Autodesk Fusion 360 part; units mm, degrees
note: some values were not read from the file. Set by a fixed rule: which sketch regions a step uses.
(part 2 of 2)
sketch "Sketch3" plane through (0, 0, 4.699) normal (0, 0, 1) x (-1, 0, 0)
  line L0 (-146.1673, -221.1104) -> (-150.3628, -221.1104)
  line L1 (-150.3628, -221.1104) -> (-150.3628, -216.6156)
  line L2 (-150.3628, -216.6156) -> (-146.1673, -216.6156)
  line L3 (-146.1673, -216.6156) -> (-146.1673, -221.1104)
  line L4 (-156.9944, -229.4223) -> (-156.9944, -223.3483)
  line L5 (-156.9944, -223.3483) -> (-152.6466, -223.3483)
  line L6 (-152.6466, -223.3483) -> (-152.6466, -229.4223)
  line L7 (-152.6466, -229.4223) -> (-156.9944, -229.4223)
  line L8 (-170.3485, -221.1104) -> (-170.3485, -216.6156)
  line L9 (-170.3485, -216.6156) -> (-165.8649, -216.6156)
  line L10 (-165.8649, -216.6156) -> (-165.8649, -221.1104)
  line L11 (-165.8649, -221.1104) -> (-170.3485, -221.1104)
  line L12 (-180.9883, -210.0039) -> (-180.9883, -214.3606)
  line L13 (-180.9883, -214.3606) -> (-183.4799, -214.3606)
  line L14 (-183.4799, -214.3606) -> (-181.7379, -210.0039)
  line L15 (-181.7379, -210.0039) -> (-180.9883, -210.0039)
  line L16 (-156.9944, -233.3153) -> (-156.9944, -231.7356)
  line L17 (-156.9944, -231.7356) -> (-154.4457, -231.7356)
  line L18 (-154.4457, -231.7356) -> (-156.9944, -233.3153)
  line L19 (-150.3628, -223.3483) -> (-146.1673, -223.3483)
  line L20 (-146.1673, -223.3483) -> (-146.1673, -226.6039)
  line L21 (-146.1673, -226.6039) -> (-150.3628, -229.2048)
  line L22 (-150.3628, -229.2048) -> (-150.3628, -223.3483)
  line L23 (-152.6466, -207.7364) -> (-156.9944, -207.7364)
  line L24 (-156.9944, -207.7364) -> (-156.9944, -203.394)
  line L25 (-156.9944, -203.394) -> (-152.6466, -203.394)
  line L26 (-152.6466, -203.394) -> (-152.6466, -207.7364)
  line L27 (-143.2758, -207.7364) -> (-143.8532, -207.7364)
  line L28 (-143.8532, -207.7364) -> (-143.8532, -206.2865)
  line L29 (-143.8532, -206.2865) -> (-143.2758, -207.7364)
  line L30 (-163.3746, -235.1382) -> (-163.3746, -231.9856)
  line L31 (-163.3746, -231.9856) -> (-159.447, -231.9856)
  line L32 (-159.447, -231.9856) -> (-159.447, -234.8356)
  line L33 (-159.447, -234.8356) -> (-161.6393, -236.1945)
  line L34 (-161.6393, -236.1945) -> (-163.3746, -235.1382)
  line L35 (-172.6153, -203.394) -> (-172.6153, -207.7364)
  line L36 (-172.6153, -207.7364) -> (-178.675, -207.7364)
  line L37 (-178.675, -207.7364) -> (-178.675, -203.394)
  line L38 (-178.675, -203.394) -> (-172.6153, -203.394)
  line L39 (-163.616, -229.4223) -> (-163.616, -223.3483)
  line L40 (-163.616, -223.3483) -> (-159.2509, -223.3483)
  line L41 (-159.2509, -223.3483) -> (-159.2509, -229.4223)
  line L42 (-159.2509, -229.4223) -> (-163.616, -229.4223)
  line L43 (-165.8649, -190.62) -> (-165.8649, -194.6061)
  line L44 (-165.8649, -194.6061) -> (-170.3485, -194.6061)
  line L45 (-170.3485, -194.6061) -> (-170.3485, -192.7692)
  line L46 (-170.3485, -192.7692) -> (-165.8649, -190.62)
  line L47 (-180.9883, -223.3483) -> (-180.9883, -224.6638)
  line L48 (-180.9883, -224.6638) -> (-183.1496, -223.3483)
  line L49 (-183.1496, -223.3483) -> (-180.9883, -223.3483)
  line L50 (-163.616, -214.3606) -> (-163.616, -210.0039)
  line L51 (-163.616, -210.0039) -> (-159.2509, -210.0039)
  line L52 (-159.2509, -210.0039) -> (-159.2509, -214.3606)
  line L53 (-159.2509, -214.3606) -> (-163.616, -214.3606)
  line L54 (-165.8649, -196.9098) -> (-165.8649, -201.1101)
  line L55 (-165.8649, -201.1101) -> (-170.3485, -201.1101)
  line L56 (-170.3485, -201.1101) -> (-170.3485, -196.9098)
  line L57 (-170.3485, -196.9098) -> (-165.8649, -196.9098)
  line L58 (-180.9883, -208.1294) -> (-180.9883, -208.2364)
  line L59 (-180.9883, -208.2364) -> (-181.031, -208.2364)
  line L60 (-181.031, -208.2364) -> (-180.9883, -208.1294)
  line L61 (-152.6466, -193.2326) -> (-152.6466, -194.6061)
  line L62 (-152.6466, -194.6061) -> (-156.9944, -194.6061)
  line L63 (-156.9944, -194.6061) -> (-156.9944, -191.0845)
  line L64 (-156.9944, -191.0845) -> (-152.6466, -193.2326)
  line L65 (-159.2509, -196.9098) -> (-159.2509, -201.1101)
  line L66 (-159.2509, -201.1101) -> (-163.616, -201.1101)
  line L67 (-163.616, -201.1101) -> (-163.616, -196.9098)
  line L68 (-163.616, -196.9098) -> (-159.2509, -196.9098)
  line L69 (-172.6153, -210.0039) -> (-172.6153, -214.3606)
  line L70 (-172.6153, -214.3606) -> (-178.675, -214.3606)
  line L71 (-178.675, -214.3606) -> (-178.675, -210.0039)
  line L72 (-178.675, -210.0039) -> (-172.6153, -210.0039)
  line L73 (-152.6466, -210.0039) -> (-152.6466, -214.3606)
  line L74 (-152.6466, -214.3606) -> (-156.9944, -214.3606)
  line L75 (-156.9944, -214.3606) -> (-156.9944, -210.0039)
  line L76 (-156.9944, -210.0039) -> (-152.6466, -210.0039)
  line L77 (-165.8649, -203.394) -> (-165.8649, -207.7364)
  line L78 (-165.8649, -207.7364) -> (-170.3485, -207.7364)
  line L79 (-170.3485, -207.7364) -> (-170.3485, -203.394)
  line L80 (-170.3485, -203.394) -> (-165.8649, -203.394)
  line L81 (-159.2509, -194.6061) -> (-163.616, -194.6061)
  line L82 (-163.616, -194.6061) -> (-163.616, -189.5422)
  line L83 (-163.616, -189.5422) -> (-161.8395, -188.6907)
  line L84 (-161.8395, -188.6907) -> (-159.2509, -189.9694)
  line L85 (-159.2509, -189.9694) -> (-159.2509, -194.6061)
  line L86 (-169.3681, -231.7356) -> (-165.8649, -231.7356)
  line L87 (-165.8649, -231.7356) -> (-165.8649, -233.8679)
  line L88 (-165.8649, -233.8679) -> (-169.3681, -231.7356)
  line L89 (-146.1673, -210.0039) -> (-146.1673, -214.3606)
  line L90 (-146.1673, -214.3606) -> (-150.3628, -214.3606)
  line L91 (-150.3628, -214.3606) -> (-150.3628, -210.0039)
  line L92 (-150.3628, -210.0039) -> (-146.1673, -210.0039)
  line L93 (-172.6153, -193.856) -> (-172.6153, -194.6061)
  line L94 (-172.6153, -194.6061) -> (-174.1802, -194.6061)
  line L95 (-174.1802, -194.6061) -> (-172.6153, -193.856)
  line L96 (-143.8532, -221.1104) -> (-143.8532, -216.6156)
  line L97 (-143.8532, -216.6156) -> (-139.739, -216.6156)
  line L98 (-139.739, -216.6156) -> (-137.9485, -221.1104)
  line L99 (-137.9485, -221.1104) -> (-143.8532, -221.1104)
  line L100 (-178.675, -216.6156) -> (-172.6153, -216.6156)
  line L101 (-172.6153, -216.6156) -> (-172.6153, -221.1104)
  line L102 (-172.6153, -221.1104) -> (-178.675, -221.1104)
  line L103 (-178.675, -221.1104) -> (-178.675, -216.6156)
  line L104 (-149.8661, -194.6061) -> (-150.3628, -194.6061)
  line L105 (-150.3628, -194.6061) -> (-150.3628, -194.3607)
  line L106 (-150.3628, -194.3607) -> (-149.8661, -194.6061)
  line L107 (-159.2509, -207.7364) -> (-163.616, -207.7364)
  line L108 (-163.616, -207.7364) -> (-163.616, -203.394)
  line L109 (-163.616, -203.394) -> (-159.2509, -203.394)
  line L110 (-159.2509, -203.394) -> (-159.2509, -207.7364)
  line L111 (-184.3821, -216.6156) -> (-180.9883, -216.6156)
  line L112 (-180.9883, -216.6156) -> (-180.9883, -221.1104)
  line L113 (-180.9883, -221.1104) -> (-186.1794, -221.1104)
  line L114 (-186.1794, -221.1104) -> (-184.3821, -216.6156)
  line L115 (-146.1673, -200.4774) -> (-146.1673, -201.1101)
  line L116 (-146.1673, -201.1101) -> (-150.3628, -201.1101)
  line L117 (-150.3628, -201.1101) -> (-150.3628, -196.9098)
  line L118 (-150.3628, -196.9098) -> (-147.5883, -196.9098)
  line L119 (-147.5883, -196.9098) -> (-146.1673, -200.4774)
  line L120 (-163.616, -216.6156) -> (-159.2509, -216.6156)
  line L121 (-159.2509, -216.6156) -> (-159.2509, -221.1104)
  line L122 (-159.2509, -221.1104) -> (-163.616, -221.1104)
  line L123 (-163.616, -221.1104) -> (-163.616, -216.6156)
  line L124 (-170.3485, -229.4223) -> (-170.3485, -223.3483)
  line L125 (-170.3485, -223.3483) -> (-165.8649, -223.3483)
  line L126 (-165.8649, -223.3483) -> (-165.8649, -229.4223)
  line L127 (-165.8649, -229.4223) -> (-170.3485, -229.4223)
  line L128 (-172.6153, -196.9098) -> (-172.6153, -201.1101)
  line L129 (-172.6153, -201.1101) -> (-178.1818, -201.1101)
  line L130 (-178.1818, -201.1101) -> (-176.5021, -196.9098)
  line L131 (-176.5021, -196.9098) -> (-172.6153, -196.9098)
  line L132 (-152.6466, -196.9098) -> (-152.6466, -201.1101)
  line L133 (-152.6466, -201.1101) -> (-156.9944, -201.1101)
  line L134 (-156.9944, -201.1101) -> (-156.9944, -196.9098)
  line L135 (-156.9944, -196.9098) -> (-152.6466, -196.9098)
  line L136 (-146.1673, -207.7364) -> (-150.3628, -207.7364)
  line L137 (-150.3628, -207.7364) -> (-150.3628, -203.394)
  line L138 (-150.3628, -203.394) -> (-146.1673, -203.394)
  line L139 (-146.1673, -203.394) -> (-146.1673, -207.7364)
  line L140 (-143.8532, -223.3483) -> (-140.9146, -223.3483)
  line L141 (-140.9146, -223.3483) -> (-143.8532, -225.1699)
  line L142 (-143.8532, -225.1699) -> (-143.8532, -223.3483)
  line L143 (-156.9944, -216.6156) -> (-152.6466, -216.6156)
  line L144 (-152.6466, -216.6156) -> (-152.6466, -221.1104)
  line L145 (-152.6466, -221.1104) -> (-156.9944, -221.1104)
  line L146 (-156.9944, -221.1104) -> (-156.9944, -216.6156)
  line L147 (-142.3724, -210.0039) -> (-140.6369, -214.3606)
  line L148 (-140.6369, -214.3606) -> (-143.8532, -214.3606)
  line L149 (-143.8532, -214.3606) -> (-143.8532, -210.0039)
  line L150 (-143.8532, -210.0039) -> (-142.3724, -210.0039)
  line L151 (-173.1698, -229.4223) -> (-178.675, -226.0716)
  line L152 (-178.675, -226.0716) -> (-178.675, -223.3483)
  line L153 (-178.675, -223.3483) -> (-172.6153, -223.3483)
  line L154 (-172.6153, -223.3483) -> (-172.6153, -229.4223)
  line L155 (-172.6153, -229.4223) -> (-173.1698, -229.4223)
  line L156 (-170.3485, -210.0039) -> (-165.8649, -210.0039)
  line L157 (-165.8649, -210.0039) -> (-165.8649, -214.3606)
  line L158 (-165.8649, -214.3606) -> (-170.3485, -214.3606)
  line L159 (-170.3485, -214.3606) -> (-170.3485, -210.0039)
  line L160 (-158.1689, -182.2481) -> (-158.1689, -111.4565)
  line L161 (-158.1689, -111.4565) -> (-158.8039, -111.4565)
  line L162 (-158.8039, -111.4565) -> (-158.8039, -106.68)
  line L163 (-158.8039, -106.68) -> (-165.1539, -106.68)
  line L164 (-165.1539, -106.68) -> (-165.1539, -111.4565)
  line L165 (-165.1539, -111.4565) -> (-165.7889, -111.4565)
  line L166 (-165.7889, -111.4565) -> (-165.7889, -182.3323)
  line L167 (-165.7889, -182.3323) -> (-168.7102, -180.8892)
  line L168 (-168.7102, -180.8892) -> (-170.2391, -183.9833)
  line L169 (-170.2391, -183.9833) -> (-165.9602, -186.0971)
  line L170 (-165.9602, -186.0971) -> (-178.2439, -192.1658)
  line L171 (-178.2439, -192.1658) -> (-180.2447, -195.7123)
  line L172 (-180.2447, -195.7123) -> (-191.2572, -223.0614)
  line L173 (-191.2572, -223.0614) -> (-194.8572, -232.3981)
  line L174 (-194.8572, -232.3981) -> (-191.7134, -233.6497)
  line L175 (-191.7134, -233.6497) -> (-188.2271, -224.8966)
  line L176 (-188.2271, -224.8966) -> (-165.345, -239.08)
  line L177 (-165.345, -239.08) -> (-167.1041, -240.1702)
  line L178 (-167.1041, -240.1702) -> (-165.2823, -243.1079)
  line L179 (-165.2823, -243.1079) -> (-162.0641, -241.1134)
  line L180 (-162.0641, -241.1134) -> (-158.8458, -243.1079)
  line L181 (-158.8458, -243.1079) -> (-157.0243, -240.1702)
  line L182 (-157.0243, -240.1702) -> (-158.7831, -239.08)
  line L183 (-158.7831, -239.08) -> (-135.9013, -224.8966)
  line L184 (-135.9013, -224.8966) -> (-132.4147, -233.6497)
  line L185 (-132.4147, -233.6497) -> (-129.2709, -232.3981)
  line L186 (-129.2709, -232.3981) -> (-132.8709, -223.0612)
  line L187 (-132.8709, -223.0612) -> (-134.3845, -219.435)
  line L188 (-134.3845, -219.435) -> (-143.8837, -195.7123)
  line L189 (-143.8837, -195.7123) -> (-145.8842, -192.1658)
  line L190 (-145.8842, -192.1658) -> (-158.1682, -186.0971)
  line L191 (-158.1682, -186.0971) -> (-153.8892, -183.9833)
  line L192 (-153.8892, -183.9833) -> (-155.4181, -180.8892)
  line L193 (-155.4181, -180.8892) -> (-158.1689, -182.2481)
equation "d2 = MaterialThickness"
equation "MaterialThickness = 0.185 in"
equation "d4 = LegNotchLength"
equation "d6 = MaterialThickness / 2"
equation "LegNotchLength = 1.5 in"
equation "BodyNotchLength = 0.5 in"
equation "d9 = LegNotchLength"
equation "d12 = BodyNotchLength"
equation "d13 = MaterialThickness"
equation "d16 = BodyNotchLength * 0.75"
equation "d17 = MaterialThickness"
equation "d18 = BodyNotchLength * 0.775"
equation "d19 = MaterialThickness"
equation "d20 = ( 1.172 * 2 ) * 1 in"
equation "d22 = SpineWidth"
equation "d23 = MaterialThickness"
equation "d24 = ( 0.194 * 2 ) * 1 in"
equation "d25 = MaterialThickness"
equation "d26 = ( 0.194 * 2 ) * 1 in"
equation "d27 = MaterialThickness"
equation "d28 = ( 1 * 2 ) * 1 in"
equation "d30 = SpineWidth"
equation "d31 = MaterialThickness"
equation "d32 = ( 0.282 * 2 ) * 1 in"
equation "d33 = MaterialThickness"
equation "d34 = ( 0.282 * 2 ) * 1 in"
equation "d35 = MaterialThickness"
equation "d36 = ( 0.903512 * 2 ) * 1 in"
equation "d38 = SpineWidth"
equation "d39 = MaterialThickness"
equation "d44 = ( 0.85 * 2 ) * 1 in"
equation "d46 = SpineWidth - 0.05 in"
equation "d47 = MaterialThickness"
equation "d48 = ( 0.219 * 2 ) * 1 in"
equation "d49 = MaterialThickness"
equation "d50 = ( 0.219 * 2 ) * 1 in"
equation "d51 = MaterialThickness"
equation "d52 = SpineWidth"
equation "SpineWidth = 0.3 in"
equation "d59 = MaterialThickness"
equation "d67 = MaterialThickness"
